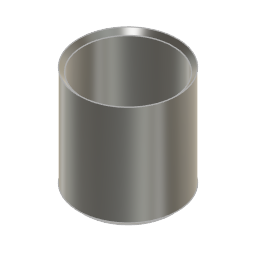
basic_potjie (Autodesk Fusion 360 design; units mm, degrees)
Autodesk Fusion 360 part; units mm, degrees
sketch "Sketch1" plane through (0, 0, 0) normal (0, 0, 1) x (1, 0, 0)
  circle A0 centre (0, 0) radius 25
  circle A1 centre (0, 0) radius 28
  dimension "d4" = 50
  dimension "d5" = 56
  constraint coincident A0.centre A1.centre
  measures "d4" diameter of A0
  measures "d5" diameter of A1
extrude "Extrude1" add sketch "Sketch1" along normal blind 3 contours A0
extrude "Extrude2" add sketch "Sketch1" along normal blind 60
chamfer "Chamfer2" distance 3 angle 45 1 edges at (-26.1052, -10.1252, 0)
move_face "OffsetFaces1" offset -0.5 1 faces at (24.8758, -2.4892, 22)
chamfer "Chamfer3" distance 3 angle 45 1 edges at (-23.7743, -9.2212, 3)
chamfer "Chamfer4" distance 2.5 angle 45 1 edges at (-23.7743, 9.2212, 60)
equation "wall_thinkness = 3 mm"
equation "pot_height = 60 mm"
equation "pot_diameter = 50 mm"
equation "d4 = pot_diameter"
equation "d5 = pot_diameter + ( 2 * wall_thinkness )"
equation "d6 = wall_thinkness"
equation "d8 = pot_height"
equation "pot_bottom_outer_fillet = 10 mm"
equation "pot_finger_cutout_num = 2"
equation "pot_finger_cutout_width = 20 mm"
equation "pot_finger_cutout_height = 7 mm"
named bodies: "simple_potjie"
